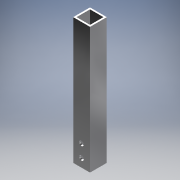
# Autodesk Inventor part: Vertical Support 1
Saved by Autodesk Inventor 2019.4 (Build 234330000, 330)
## iProperties
Created: 2020-01-19
Part Number: Vertical Support 1
Material: Aluminum 6061
Document SubType Name: Modeling
Designer: Mark
Mass: 58.32 g
Surface Area: 218.88 cm^2
Volume: 21.6 cm^3
Density: 2.7 g/cm^3
Appearance: Aluminum - Flat
Author: Mark
Autodesk Inventor part; units mm, degrees
ref_plane "YZ Plane" through (0, 0, 0) normal (1, 0, 0) x (0, 1, 0)
ref_plane "XZ Plane" through (0, 0, 0) normal (0, 1, 0) x (-1, 0, 0)
ref_plane "XY Plane" through (0, 0, 0) normal (0, 0, 1) x (1, 0, 0)
sketch "Sketch1" plane through (0, 0, 0) normal (0, 1, 0) x (-1, 0, 0)
  line L0 (-10, 10) -> (10, 10)
  line L1 (10, 10) -> (10, -10)
  line L2 (10, -10) -> (-10, -10)
  line L3 (-10, -10) -> (-10, 10)
  line L4 (-10, 10) -> (10, -10) construction
  line L5 (10, 10) -> (-10, -10) construction
  line L6 (-8, 8) -> (8, 8)
  line L7 (8, 8) -> (8, -8)
  line L8 (8, -8) -> (-8, -8)
  line L9 (-8, -8) -> (-8, 8)
  line L10 (-8, 8) -> (8, -8) construction
  line L11 (8, 8) -> (-8, -8) construction
  point P0 (0, 0)
  dimension "d0" = 20
  dimension "d1" = 20
  dimension "d2" = 16
  dimension "d3" = 16
  constraints: 24 end point, 4 midpoint, 4 parallel, 2 horizontal, 2 perpendicular
  measures "d0" distance of L1.end L2.end
  measures "d1" distance of L0.end L1.end
  measures "d2" distance of L7.end L8.end
  measures "d3" distance of L6.end L7.end
extrude "Extrusion1" add sketch "Sketch1" along normal blind 150
sketch "Sketch2" plane through (-10, 0, 10) normal (0, 0, 1) x (1, 0, 0)
  circle A0 centre (10, 10) radius 2.75
  circle A1 centre (10, 25) radius 2.75
  line L0 (20, 0) -> (20, 150) projected
  line L1 (20, 0) -> (0, 0) projected
  circle A2 centre (10, 140) radius 2.75
  circle A3 centre (10, 119.5) radius 2.75
  line L2 (0, 0) -> (0, 150) projected
  line L3 (0, 150) -> (20, 150) projected
  point P0 (10, 0)
  dimension "d6" = 5.5
  dimension "d7" = 5.5
  dimension "d8" = 10
  dimension "d9" = 10
  dimension "d10" = 10
  dimension "d11" = 15
  dimension "d22" = 5.5
  dimension "d23" = 5.5
  dimension "d24" = 10
  dimension "d25" = 10
  dimension "d26" = 15
  dimension "d27" = 10
  constraints: 4 centre point
  measures "d6" diameter of A0
  measures "d7" diameter of A1
  measures "d8" distance from line of L0 A1.centre
  measures "d9" distance from line of L0 A0.centre
  measures "d10" distance from line of L1 A0.centre
  measures "d11" distance of A0.centre A1.centre
  measures "d22" diameter of A2
  measures "d23" diameter of A3
  measures "d24" distance from line of L0 A2.centre
  measures "d25" distance from line of L2 A3.centre
  measures "d27" distance from line of L3 A2.centre
extrude "Extrusion2" cut sketch "Sketch2" against normal blind 20 contours A0 | A1 | A2 | A3
sketch "Sketch3" plane through (-10, 0, -10) normal (-1, 0, 0) x (0, 0, 1)
  circle A0 centre (10, 40) radius 2.75
  circle A1 centre (10, 110) radius 2.75
  line L0 (0, 150) -> (20, 150) projected
  line L1 (20, 0) -> (20, 150) projected
  line L2 (20, 0) -> (0, 0) projected
  point P0 (10, 0)
  dimension "d14" = 5.5
  dimension "d15" = 5.5
  dimension "d16" = 40
  dimension "d17" = 10
  dimension "d18" = 40
  dimension "d19" = 10
  constraints: 2 centre point
  measures "d14" diameter of A0
  measures "d15" diameter of A1
  measures "d16" distance from line of L0 A1.centre
  measures "d17" distance from line of L1 A1.centre
  measures "d18" distance from line of L2 A0.centre
  measures "d19" distance from line of L1 A0.centre
extrude "Extrusion3" cut sketch "Sketch3" against normal blind 20
body "Solid1"
